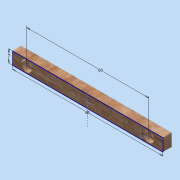
# Autodesk Inventor part: Rail
Saved by Autodesk Inventor 2015 (Build 190159000, 159)
## iProperties
Created: 2015-01-31
Part Number: Rail
Material: Wood (Birch)
Document SubType Name: Modeling
Designer: Openlab
Density: 0.55 g/cm^3
Appearance: Birch - Natural Polished
Author: Openlab
Autodesk Inventor part; units mm, degrees
ref_plane "YZ Plane" through (0, 0, 0) normal (1, 0, 0) x (0, 1, 0)
ref_plane "XZ Plane" through (0, 0, 0) normal (0, 1, 0) x (-1, 0, 0)
ref_plane "XY Plane" through (0, 0, 0) normal (0, 0, 1) x (1, 0, 0)
sketch "Sketch1" plane through (0, 0, 0) normal (0, 1, 0) x (-1, 0, 0)
  line L0 (0, 0) -> (85, 0)
  line L1 (85, 0) -> (85, -7)
  line L2 (85, -7) -> (0, -7)
  line L3 (0, -7) -> (0, 0)
  line L4 (42.5, 3) -> (42.5, -16) construction
  line L5 (45, -3.5) -> (39, -3.5) construction
  point P0 (77, -3.5)
  point P1 (8, -3.5)
  dimension "d0" = 85
  dimension "d1" = 7
  dimension "d2" = 69
  dimension "d12" = 3.5
  constraints: 12 end point, 2 horizontal, 2 parallel, 1 perpendicular, 1 symmetric about line, 1 vertical, 2 other
  measures "d0" distance of L1.end L2.end
  measures "d1" distance of L0.end L1.end
  measures "d2" distance of point (8, -3.5) point (77, -3.5)
  measures "d12" distance from line of L2 point (8, -3.5)
extrude "Extrusion1" add sketch "Sketch1" along normal blind 5
hole "Hole1" at (-77, 0, -3.5) at (-8, 0, -3.5) direction (0, 1, 0) diameter 3 end through all counterbore diameter 6 counterbore depth 2.5
body "Solid1"
